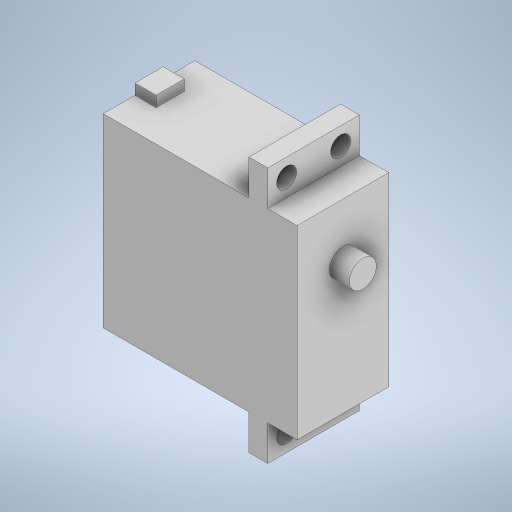
# Autodesk Inventor part: servo motor
Saved by Autodesk Inventor 2023.2 (Build 272271000, 271)
## iProperties
Created: 2023-02-10
Part Number: servo motor
Material: Generic
Document SubType Name: Modeling
Designer: Noah Postema
Density: 1 g/cm^3
Appearance: Default
Author: Noah Postema
Autodesk Inventor part; units mm, degrees
ref_plane "YZ Plane" through (0, 0, 0) normal (1, 0, 0) x (0, 1, 0)
ref_plane "XZ Plane" through (0, 0, 0) normal (0, 1, 0) x (-1, 0, 0)
ref_plane "XY Plane" through (0, 0, 0) normal (0, 0, 1) x (1, 0, 0)
sketch "Sketch1" plane through (0, 0, 0) normal (0, 0, 1) x (1, 0, 0)
  line L0 (-23.2014, 27.686) -> (18.7086, 27.686)
  line L1 (18.7086, 20.066) -> (18.7086, -20.066)
  line L2 (18.7086, -27.686) -> (-23.2014, -27.686)
  line L3 (-23.2014, -22.352) -> (-23.2014, 22.352)
  line L4 (18.7086, 0) -> (0, 0)
  line L5 (-23.2014, 22.352) -> (-18.6294, 22.352)
  line L6 (-18.6294, -22.352) -> (-23.2014, -22.352)
  line L7 (18.7086, 20.066) -> (12.3586, 20.066)
  line L8 (8.2946, 20.066) -> (-18.6294, 20.066)
  line L9 (8.2946, 27.686) -> (8.2946, 20.066)
  line L10 (8.2946, -20.066) -> (8.2946, -27.686)
  line L11 (12.3586, 27.686) -> (12.3586, 20.066)
  line L12 (12.3586, -20.066) -> (12.3586, -27.686)
  line L13 (18.7086, -20.066) -> (12.3586, -20.066)
  line L14 (8.2946, -20.066) -> (-18.6294, -20.066)
  line L15 (-18.6294, 22.352) -> (-18.6294, 20.066)
  line L16 (-18.6294, -20.066) -> (-18.6294, -22.352)
  dimension "d0" = 41.91
  dimension "d1" = 55.372
  dimension "d7" = 44.704
  constraints: 34 end point, 16 perpendicular, 6 parallel, 3 point on line, 2 horizontal, 1 midpoint, 1 other
  measures "d0" distance of L2.start L2.end
  measures "d1" distance of L0.end L2.start
  measures "d7" distance between parallel lines of L6 L5
extrude "Extrusion1" add sketch "Sketch1" along normal mid plane 19.812
sketch "Sketch2" plane through (18.7086, -20.066, 9.906) normal (1, 0, 0) x (0, 0, -1)
  line L0 (19.812, 40.132) -> (0, 40.132) projected
  circle A0 centre (9.906, 28.321) radius 2.921
  line L1 (9.906, 28.321) -> (9.906, 25.4)
  point P0 (9.906, 20.066)
  point P1 (9.906, 40.132)
  dimension "d10" = 5.842
  dimension "d11" = 14.732
  constraints: 2 end point, 1 midpoint, 1 vertical, 1 vertical alignment, 2 other
  measures "d11" distance of L1.end point (9.906, 40.132)
extrude "Extrusion2" add sketch "Sketch2" along normal blind 4.318
sketch "Sketch3" plane through (12.3586, 20.066, 9.906) normal (1, 0, 0) x (0, 0, -1)
  circle A0 centre (15.748, 3.7795) radius 2.159
  line L0 (19.812, 7.62) -> (19.812, 0) projected
  line L1 (19.812, -47.752) -> (0, -47.752) projected
  line L2 (19.812, 7.62) -> (0, 7.62) projected
  line L3 (0, -40.132) -> (0, 0) projected
  line L4 (0, -20.066) -> (19.812, -20.066) construction
  line L5 (19.812, 0) -> (19.812, -40.132) projected
  line L6 (9.906, 7.62) -> (9.906, -47.752) construction
  circle A1 centre (15.748, -43.9115) radius 2.159
  circle A2 centre (4.064, 3.7795) radius 2.159
  circle A3 centre (4.064, -43.9115) radius 2.159
  point P0 (9.906, -20.066)
  dimension "d14" = 4.064
  dimension "d15" = 4.318
  dimension "d16" = 55.372
  constraints: 4 centre point, 4 end point, 4 midpoint, 3 symmetric about line, 3 other
  measures "d14" distance from line of A0.centre L0
  measures "d15" diameter of A0
  measures "d16" distance between parallel lines of L1 L2
extrude "Extrusion3" cut sketch "Sketch3" against normal up to surface (4.064 mm away)
sketch "Sketch4" plane through (-18.6294, 20.066, 9.906) normal (1, 0, 0) x (0, 0, -1)
  line L0 (19.812, -42.418) -> (19.812, 2.286) projected
  line L1 (19.812, 2.286) -> (0, 2.286) projected
  line L2 (6.858, 2.286) -> (6.858, -42.418)
  line L3 (0, 2.286) -> (0, -42.418) projected
  line L4 (12.954, 2.286) -> (12.954, -42.418)
  line L5 (19.812, -42.418) -> (0, -42.418) projected
  line L6 (0, 0) -> (19.812, 0) projected
  line L7 (19.812, 0) -> (0, 0) projected
  line L8 (19.812, -40.132) -> (0, -40.132) projected
  line L9 (19.812, -40.132) -> (0, -40.132) projected
  point P0 (9.906, -20.066)
  point P1 (12.954, -40.132)
  point P2 (6.858, -40.132)
  point P3 (12.954, 0)
  point P4 (6.858, 0)
  dimension "d19" = 12.954
  dimension "d20" = 12.954
  constraints: 4 end point, 2 point on line, 2 vertical
  measures "d19" distance between parallel lines of L2 L0
  measures "d20" distance between parallel lines of L3 L4
extrude "Extrusion4" cut sketch "Sketch4" against normal through all contours L5 L4 L8 L0 | L6 L4 L1 L0 | L5 L3 L8 L2 | L6 L3 L1 L2
body "Solid1"
